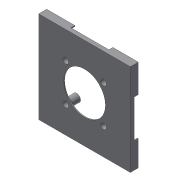
# Autodesk Inventor part: motor_mount_base2_template
Saved by Autodesk Inventor 2017 (Build 210142000, 142)
## iProperties
Created: 2018-10-29
Part Number: motor_mount_base2_template
Material: Generic
Document SubType Name: Modeling
Designer: mfans
Density: 1 g/cm^3
Appearance: Default
Author: mfans
Autodesk Inventor part; units mm, degrees
ref_plane "YZ Plane" through (0, 0, 0) normal (1, 0, 0) x (0, 1, 0)
ref_plane "XZ Plane" through (0, 0, 0) normal (0, 1, 0) x (-1, 0, 0)
ref_plane "XY Plane" through (0, 0, 0) normal (0, 0, 1) x (1, 0, 0)
sketch "Sketch1" plane through (0, 0, 0) normal (0, 1, 0) x (-1, 0, 0)
  line L0 (45, 45) -> (-45, 45)
  line L1 (-45, 45) -> (-45, -45)
  line L2 (-45, -45) -> (45, -45)
  line L3 (45, -45) -> (45, 45)
  line L4 (45, 45) -> (-45, -45) construction
  line L5 (-45, 45) -> (45, -45) construction
  line L6 (-46, 46) -> (46, 46)
  line L7 (46, 46) -> (46, -46)
  line L8 (46, -46) -> (-46, -46)
  line L9 (-46, -46) -> (-46, 46)
  line L10 (-46, 46) -> (46, -46) construction
  line L11 (46, 46) -> (-46, -46) construction
  point P0 (0, 0)
  dimension "d0" = 90
  dimension "d1" = 90
  dimension "d2" = 92
  dimension "d3" = 92
  constraints: 24 end point, 4 midpoint, 4 parallel, 2 horizontal, 2 perpendicular
  measures "d0" distance of L2.end L1.end
  measures "d1" distance of L0.end L1.end
  measures "d2" distance of L7.end L8.end
  measures "d3" distance of L8.end L6.start
extrude "Extrusion1" add sketch "Sketch1" along normal blind 1 contours L3 L2 L1 L0 | L6 L7 L8 L9
sketch "Sketch2" plane through (0, 1, 0) normal (0, 1, 0) x (1, 0, 0)
  line L0 (-46, -46) -> (46, -46) projected
  line L1 (46, -46) -> (46, 46) projected
  line L2 (46, 46) -> (-46, 46) projected
  line L3 (-46, 46) -> (-46, -46) projected
  line L4 (45, 45) -> (-45, 45)
  line L5 (-45, -20.5) -> (-45, -45)
  line L6 (-45, -45) -> (-17.75, -45)
  line L7 (45, -45) -> (45, 45)
  line L8 (45, 45) -> (-45, -45) construction
  line L9 (-45, 45) -> (45, -45) construction
  line L10 (-27.75, -30.5) -> (-17.75, -30.5)
  line L11 (-17.75, -30.5) -> (-17.75, -29.5)
  line L12 (-17.75, -29.5) -> (-27.75, -29.5)
  line L13 (-27.75, -29.5) -> (-27.75, -30.5)
  line L14 (-27.75, -30.5) -> (-26.75, -30.5)
  line L15 (-26.75, -30.5) -> (-26.75, -20.5)
  line L16 (-26.75, -20.5) -> (-27.75, -20.5)
  line L17 (-27.75, -20.5) -> (-27.75, -30.5)
  line L18 (-17.75, -45) -> (-17.75, -46)
  line L19 (-46, -46) -> (46, -46) projected
  line L20 (-45, -20.5) -> (-46, -20.5)
  point P0 (0, 0)
  dimension "d6" = 90
  dimension "d7" = 90
  dimension "d8" = 1
  dimension "d9" = 1
  dimension "d10" = 10
  dimension "d11" = 10
  dimension "d12" = 14.5
  dimension "d13" = 17.25
  constraints: 32 end point, 6 parallel, 4 perpendicular, 3 horizontal, 2 midpoint, 2 point on line, 1 vertical
  measures "d6" distance of L5.end L7.start
  measures "d7" distance of L4.end L5.end
  measures "d8" distance of L15.end L16.end
  measures "d9" distance of L10.end L11.end
  measures "d10" distance of L11.end L12.end
  measures "d11" distance of L14.end L15.end
  measures "d12" distance between parallel lines of L6 L10
  measures "d13" distance between parallel lines of L5 L17
sketch "Sketch3" plane through (0, 1, 0) normal (0, 1, 0) x (1, 0, 0)
  line L0 (-27.75, -30.5) -> (-17.75, -30.5) projected
  line L1 (-27.75, -20.5) -> (-27.75, -30.5) projected
  line L2 (-26.75, -30.5) -> (-26.75, -20.5) projected
  line L3 (-17.75, -29.5) -> (-27.75, -29.5) projected
  line L4 (-26.75, -20.5) -> (-27.75, -20.5) projected
  line L5 (-17.75, -45) -> (-17.75, -46) projected
  line L6 (-45, -20.5) -> (-46, -20.5) projected
  line L7 (-46, 46) -> (-46, -46) projected
  line L8 (-45, -20.5) -> (-46, -20.5)
  line L9 (-46, -20.5) -> (-46, -46)
  line L10 (-46, -46) -> (-45, -46)
  line L11 (-45, -46) -> (-45, -20.5)
  line L12 (-46, -46) -> (46, -46) projected
  line L13 (-46, -46) -> (-17.75, -46)
  line L14 (-17.75, -46) -> (-17.75, -45)
  line L15 (-17.75, -45) -> (-46, -45)
  line L16 (-46, -45) -> (-46, -46)
  line L17 (-27.75, -30.5) -> (-17.75, -30.5)
  line L18 (-17.75, -30.5) -> (-17.75, -29.5)
  line L19 (-17.75, -29.5) -> (-27.75, -29.5)
  line L20 (-27.75, -29.5) -> (-27.75, -30.5)
  point P0 (0, 0)
  constraints: 24 end point, 6 parallel, 3 horizontal, 3 perpendicular
extrude "Extrusion2" add sketch "Sketch3" along normal blind 7
sketch "Sketch4" plane through (-45, 1, 20.5) normal (0, 0, -1) x (-1, 0, 0)
  line L0 (-17.25, 0) -> (-18.25, 0) projected
  line L1 (-17.25, 0) -> (-17.25, 7) projected
  line L2 (-18.25, 7) -> (-17.25, 7) projected
  line L3 (-18.25, 0) -> (-18.25, 7) projected
  line L4 (1, 0) -> (0, 0) projected
  line L5 (1, 0) -> (1, 7) projected
  line L6 (0, 7) -> (1, 7) projected
  line L7 (0, 0) -> (0, 7) projected
  line L8 (0, 0) -> (-27.25, 0) projected
  arc A0 (-17.25, 4.027) -> (0, 4.027) centre (-8.625, 11.25) ccw
  line L9 (-91, 0) -> (1, 0) projected
  line L10 (-17.25, 0) -> (-17.25, 7) projected
  line L11 (-8.625, 0) -> (-17.25, 0)
  line L12 (-17.25, 0) -> (-17.25, 4.027)
  line L13 (0, 0) -> (0, 7) projected
  line L14 (-8.625, 0) -> (0, 0)
  line L15 (0, 0) -> (0, 4.027)
  point P0 (-45, -1)
  dimension "d16" = 22.5
  dimension "d17" = 8.625
  constraints: 8 end point, 3 point on circle, 3 point on line, 1 centre point, 1 tangent
  measures "d16" diameter of A0
  measures "d17" distance from line of L1 A0.centre
extrude "Extrusion3" add sketch "Sketch4" against normal blind 10 contours A0 L7 L8 | L1 A0 L8
sketch "Sketch5" plane through (0, 1, 0) normal (0, 1, 0) x (1, 0, 0)
  line L0 (-17.75, -46) -> (46, -46) projected
  line L1 (-46, -20.5) -> (-46, -46) projected
  point P0 (0, 0)
  point P1 (-19, -19)
  dimension "d23" = 27
  dimension "d24" = 27
  measures "d23" distance from line of L0 point (-19, -19)
  measures "d24" distance from line of L1 point (-19, -19)
hole "Hole1" at (-19, 1, 19) direction (0, -1, 0) diameter 4 end through all
pattern_circular "Circular Pattern2" count 4 over 360 about axis through (0, -10, 0) along (0, 1, 0) of "Extrusion2", "Extrusion3", "Hole1"
sketch "Sketch6" plane through (0, 1, 0) normal (0, 1, 0) x (1, 0, 0)
  circle A0 centre (0, 0) radius 21
  dimension "d35" = 42
  constraints: 1 centre point, 1 coincident
  measures "d35" diameter of A0
extrude "Extrusion4" cut sketch "Sketch6" against normal blind 10
sketch "Sketch7" plane through (0, 1, 0) normal (0, 1, 0) x (1, 0, 0)
  line L0 (45, 45) -> (-45, 45)
  line L1 (-45, 45) -> (-45, -45)
  line L2 (-45, -45) -> (45, -45)
  line L3 (45, -45) -> (45, 45)
  line L4 (45, 45) -> (-45, -45) construction
  line L5 (-45, 45) -> (45, -45) construction
  line L6 (46, -46) -> (-46, -46) projected
  line L7 (-46, 46) -> (46, 46)
  line L8 (46, 46) -> (46, -46)
  line L9 (46, -46) -> (-46, -46)
  line L10 (-46, -46) -> (-46, 46)
  line L11 (-46, 46) -> (46, -46) construction
  line L12 (46, 46) -> (-46, -46) construction
  point P0 (0, 0)
  dimension "d38" = 90
  dimension "d39" = 90
  constraints: 24 end point, 4 midpoint, 4 parallel, 2 horizontal, 2 perpendicular
  measures "d38" distance of L2.end L1.end
  measures "d39" distance of L2.end L0.start
extrude "Extrusion5" add sketch "Sketch7" along normal blind 3
sketch "Sketch8" plane through (0, 1, 0) normal (0, 1, 0) x (1, 0, 0)
  circle A0 centre (-19, -19) radius 2 projected
  circle A1 centre (19, -19) radius 2 projected
  circle A2 centre (19, 19) radius 2 projected
  circle A3 centre (-19, 19) radius 2 projected
  circle A4 centre (0, 0) radius 21 projected
  line L0 (-45, -45) -> (20.5, -45) projected
  line L1 (20.5, -45) -> (20.5, -36.375) projected
  line L2 (20.5, -36.375) -> (20.5, -26.75) projected
  line L3 (20.5, -26.75) -> (29.5, -26.75) projected
  line L4 (29.5, -26.75) -> (29.5, -17.75) projected
  line L5 (29.5, -17.75) -> (30.5, -17.75) projected
  line L6 (30.5, -17.75) -> (30.5, -36.375) projected
  line L7 (30.5, -36.375) -> (30.5, -45) projected
  line L8 (30.5, -45) -> (45, -45) projected
  line L9 (45, -45) -> (45, 20.5) projected
  line L10 (45, 20.5) -> (36.375, 20.5) projected
  line L11 (36.375, 20.5) -> (26.75, 20.5) projected
  line L12 (26.75, 20.5) -> (26.75, 29.5) projected
  line L13 (26.75, 29.5) -> (17.75, 29.5) projected
  line L14 (17.75, 29.5) -> (17.75, 30.5) projected
  line L15 (17.75, 30.5) -> (36.375, 30.5) projected
  line L16 (36.375, 30.5) -> (45, 30.5) projected
  line L17 (45, 30.5) -> (45, 45) projected
  line L18 (45, 45) -> (-20.5, 45) projected
  line L19 (-20.5, 45) -> (-20.5, 36.375) projected
  line L20 (-20.5, 36.375) -> (-20.5, 26.75) projected
  line L21 (-20.5, 26.75) -> (-29.5, 26.75) projected
  line L22 (-29.5, 26.75) -> (-29.5, 17.75) projected
  line L23 (-29.5, 17.75) -> (-30.5, 17.75) projected
  line L24 (-30.5, 17.75) -> (-30.5, 36.375) projected
  line L25 (-30.5, 36.375) -> (-30.5, 45) projected
  line L26 (-30.5, 45) -> (-45, 45) projected
  line L27 (-45, 45) -> (-45, -20.5) projected
  line L28 (-45, -20.5) -> (-36.375, -20.5) projected
  line L29 (-36.375, -20.5) -> (-26.75, -20.5) projected
  line L30 (-26.75, -20.5) -> (-26.75, -29.5) projected
  line L31 (-26.75, -29.5) -> (-17.75, -29.5) projected
  line L32 (-17.75, -29.5) -> (-17.75, -30.5) projected
  line L33 (-17.75, -30.5) -> (-36.375, -30.5) projected
  line L34 (-36.375, -30.5) -> (-45, -30.5) projected
  line L35 (-45, -30.5) -> (-45, -45) projected
  circle A5 centre (-19, -19) radius 2 projected
  circle A6 centre (-19, -19) radius 4
  dimension "d42" = 8
  constraints: 1 centre point, 1 coincident
  measures "d42" diameter of A6
extrude "Extrusion6" add sketch "Sketch8" along normal blind 10 contours A6
sketch "Sketch9" plane through (0, 0, 0) normal (0, -1, 0) x (1, 0, 0)
  circle A0 centre (0, 0) radius 21 projected
  circle A1 centre (-19, -19) radius 2 projected
  circle A2 centre (19, -19) radius 2 projected
  circle A3 centre (19, 19) radius 2 projected
  circle A4 centre (-19, 19) radius 2 projected
  line L0 (46, 46) -> (-46, 46) projected
  line L1 (-46, 46) -> (-46, -46) projected
  line L2 (-46, -46) -> (46, -46) projected
  line L3 (46, -46) -> (46, 46) projected
  circle A5 centre (-19, 19) radius 3
  dimension "d45" = 6
  constraints: 1 centre point, 1 coincident
  measures "d45" diameter of A5
extrude "Extrusion7" cut sketch "Sketch9" against normal blind 10 contours A5
fillet "Fillet1" radius 2 1 edges at (-23, 1, 19)
pattern_circular "Circular Pattern3" count 4 over 360 about axis through (0, -10, 0) along (0, 1, 0) of "Extrusion6", "Extrusion7", "Fillet1"
body "Solid1"
